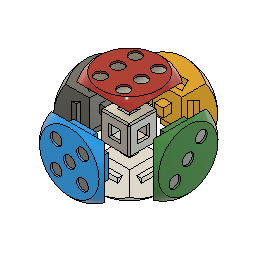
kostka v14 (Autodesk Fusion 360 design; units mm, degrees)
Autodesk Fusion 360 part; units mm, degrees
sketch "Sketch1" plane through (0, 0, 0) normal (0, 0, 1) x (1, 0, 0)
  line L0 (12, -12) -> (-12, -12)
  line L1 (-12, -12) -> (-12, 12)
  line L2 (-12, 12) -> (12, 12)
  line L3 (12, 12) -> (12, -12)
  line L4 (12, -12) -> (-12, 12) construction
  line L5 (-12, -12) -> (12, 12) construction
  line L6 (-5, -5) -> (5, -5)
  line L7 (5, -5) -> (5, 5)
  line L8 (5, 5) -> (-5, 5)
  line L9 (-5, 5) -> (-5, -5)
  line L10 (-5, -5) -> (5, 5) construction
  line L11 (5, -5) -> (-5, 5) construction
  dimension "d1" = 24
  dimension "d2" = 24
  dimension "d6" = 10
  dimension "d7" = 10
  constraint horizontal L0
  constraint perpendicular L0 L1
  constraint parallel L0 L2
  constraint parallel L1 L3
  constraint coincident L4 origin
  constraint coincident L5 origin
  constraint horizontal L6
  constraint perpendicular L6 L7
  constraint parallel L6 L8
  constraint parallel L7 L9
  constraint coincident L10 origin
  constraint coincident L11 origin
  measures "d1" distance of L1.end L2.end
  measures "d2" distance of L0.end L1.end
  measures "d6" distance of L7.end L8.end
  measures "d7" distance of L6.end L7.end
extrude "Extrude1" add sketch "Sketch1" along normal mid plane 24 makes body 1
ref_plane "WorkPlane1" through (-12, -12, -12) normal (0.707107, -0.707107, 0) x (0.707107, 0.707107, 0)
ref_plane "WorkPlane2" through (12, -12, -12) normal (-0.707107, -0.707107, 0) x (0.707107, -0.707107, 0)
ref_plane "WorkPlane3" through (12, -12, -12) normal (0, -0.707107, 0.707107) x (1, 0, 0)
ref_plane "WorkPlane4" through (12, -12, 12) normal (0, 0.707107, 0.707107) x (-1, 0, 0)
sphere "SpherePrimitive1" add diameter 31.5 placed x (1, 0, 0) y (0, 1, 0) z (0, 0, 1) at (0, 0, 0) separate body makes body 2
combine "Combine1" operation intersect target body 1 tool bodies 2 keep tools
split "Split1" by plane through (12, -12, 12) normal (0, 0.707107, 0.707107) bodies 1 makes body 3 at (9.4212, 10.076, -7.6011)
split "Split2" by plane through (12, -12, -12) normal (0, -0.707107, 0.707107) bodies 1 makes body 4 at (-2.4987, -12, 0.2541)
split "Split3" by plane through (-12, -12, -12) normal (0.707107, -0.707107, 0) bodies 4 makes body 5 at (-2.4987, -12, 0.2541)
split "Split4" by plane through (12, -12, -12) normal (-0.707107, -0.707107, 0) bodies 5 makes body 6 at (-2.4987, -12, 0.2541)
ref_plane "WorkPlane5" through (0, -8, 0) normal (0, 1, 0) x (-1, 0, 0)
sketch "Sketch7" plane through (0, -8, 0) normal (0, 1, 0) x (1, 0, 0)
  line L0 (4, -8) -> (-4, -8)
  line L1 (-4, -8) -> (-4, -6)
  line L2 (-4, -6) -> (4, -6)
  line L3 (4, -6) -> (4, -8)
  line L4 (4, -8) -> (-4, -6) construction
  line L5 (-4, -8) -> (4, -6) construction
  line L6 (6, -4) -> (6, 4)
  line L7 (6, 4) -> (8, 4)
  line L8 (8, 4) -> (8, -4)
  line L9 (8, -4) -> (6, -4)
  line L10 (4, 6) -> (-4, 6)
  line L11 (-4, 6) -> (-4, 8)
  line L12 (-4, 8) -> (4, 8)
  line L13 (4, 8) -> (4, 6)
  line L14 (-6, 4) -> (-6, -4)
  line L15 (-6, -4) -> (-8, -4)
  line L16 (-8, -4) -> (-8, 4)
  line L17 (-8, 4) -> (-6, 4)
  line L18 (1.5, -1.5) -> (-1.5, -1.5)
  line L19 (-1.5, -1.5) -> (-1.5, 1.5)
  line L20 (-1.5, 1.5) -> (1.5, 1.5)
  line L21 (1.5, 1.5) -> (1.5, -1.5)
  line L22 (1.5, -1.5) -> (-1.5, 1.5) construction
  line L23 (-1.5, -1.5) -> (1.5, 1.5) construction
  point P0 (0, -7)
  dimension "d9" = 8
  dimension "d10" = 2
  dimension "d12" = 360
  dimension "d15" = 7
  dimension "d70" = 3
  dimension "d71" = 3
  constraint horizontal L0
  constraint perpendicular L0 L1
  constraint parallel L0 L2
  constraint parallel L1 L3
  constraint coincident L4 P0
  constraint coincident L5 P0
  constraint horizontal L18
  constraint perpendicular L18 L19
  constraint parallel L18 L20
  constraint parallel L19 L21
  constraint coincident L22 origin
  constraint coincident L23 origin
  measures "d9" distance of L1.end L2.end
  measures "d10" distance of L0.end L1.end
  measures "d15" distance of origin P0
  measures "d70" distance of L19.end L20.end
  measures "d71" distance of L18.end L19.end
extrude "Extrude4" add sketch "Sketch7" along normal blind 6 contours L18 L19 L20 L21 bodies 6
extrude "Extrude3" cut sketch "Sketch7" along normal through all contours L10 L11 L12 L13 | L14 L15 L16 L17 bodies 6
extrude "Extrude2" add sketch "Sketch7" along normal blind 1.5 contours L0 L1 L2 L3 | L6 L7 L8 L9 bodies 6
move_face "OffsetFaces1" offset -0.03 4 faces at (9.037, -9.037, -0.3588) (-0.3588, -9.037, -9.037) (-9.037, -9.037, 0.3588) (0.3588, -9.037, 9.037) on bodies 6
move_face "OffsetFaces3" offset -0.05 8 faces at (-6.6525, -8, 1.3333) (-6.7391, -7.5, 4) (-6, -7.5, -1.3333) (-6.7391, -7.5, -4) (1.3333, -7.5, -6) (1.3333, -8, -7.305) (4, -7.5, -6.7391) (-4, -7.5, -6.7391) on bodies 6
copy_body "CopyPasteBodies1" bodies 6 makes body 7
move_body "Move1" bodies 7 to x (1, 0, 0) y (0, -1, 0) z (0, 0, -1) at (0, 0, 0)
copy_body "CopyPasteBodies2" bodies 6 makes body 8
move_body "Move2" bodies 8 to x (0, -1, 0) y (0, 0, -1) z (1, 0, 0) at (0, 0, 0)
copy_body "CopyPasteBodies3" bodies 6 makes body 9
move_body "Move3" bodies 9 to x (1, 0, 0) y (0, 0, 1) z (0, -1, 0) at (0, 0, 0)
copy_body "CopyPasteBodies4" bodies 6 makes body 10
move_body "Move4" bodies 10 to x (0, -1, 0) y (1, 0, 0) z (0, 0, 1) at (0, 0, 0)
copy_body "CopyPasteBodies5" bodies 6 makes body 11
move_body "Move5" bodies 11 to x (0, 1, 0) y (-1, 0, 0) z (0, 0, 1) at (0, 0, 0)
copy_body "Body->Comp1" bodies 6 removing the originals makes body 12 in component "No1"
copy_body "Body->Comp2" bodies 7 removing the originals makes body 13 in component "No6"
copy_body "Body->Comp3" bodies 8 removing the originals makes body 14 in component "No5"
copy_body "Body->Comp4" bodies 9 removing the originals makes body 15 in component "No2"
copy_body "Body->Comp5" bodies 10 removing the originals makes body 16 in component "No4"
copy_body "Body->Comp6" bodies 11 removing the originals makes body 17 in component "No3"
move_face "MoveFace1" to x (1, 0, 0) y (0, 0, -1) z (0, 1, 0) at (0, 0, 0) 1 faces at (12, -1.0078, -1.1876) on bodies 17 in component "No3"
sketch "Sketch1 (2)" plane through (0, 12, 0) normal (0, 1, 0) x (-1, 0, 0) in component "No6"
  circle A0 centre (0, 0) radius 10.2011
  circle A1 centre (0, 0) radius 2 construction
  circle A2 centre (-6, -4) radius 2
  circle A3 centre (0, -4) radius 2
  circle A4 centre (6, -4) radius 2
  circle A5 centre (-6, 4) radius 2
  circle A6 centre (0, 4) radius 2
  circle A7 centre (6, 4) radius 2
  dimension "d27" = 4
  dimension "d30" = 6
  dimension "d31" = 4
  constraint coincident A0.centre A1.centre
  measures "d27" diameter of A1
extrude "Extrude2'" cut sketch "Sketch1 (2)" against normal blind 0.6 contours A2 | A3 | A4 | A5 | A6 | A7 bodies 13 in component "No6"
sketch "Sketch1 (3)" plane through (0, -12, 0) normal (0, -1, 0) x (1, 0, 0) in component "No1"
  circle A0 centre (0, 0) radius 10.2011
  circle A1 centre (0, 0) radius 2
  dimension "d37" = 4
  constraint coincident A0.centre A1.centre
  measures "d37" diameter of A1
extrude "Extrude1'" cut sketch "Sketch1 (3)" against normal blind 0.6 contours A1 bodies 12 in component "No1"
sketch "Sketch1 (4)" plane through (0, 0, 12) normal (0, 0, 1) x (1, 0, 0) in component "No5"
  circle A0 centre (0, 0) radius 10.2011
  circle A1 centre (0, 0) radius 2
  circle A2 centre (-4.5255, 4.5255) radius 2
  line L0 (0, 0) -> (-6.7167, 6.7167) construction
  line L1 (0, 0) -> (-11, 0) construction
  circle A3 centre (-4.5255, -4.5255) radius 2
  circle A4 centre (4.5255, -4.5255) radius 2
  circle A5 centre (4.5255, 4.5255) radius 2
  dimension "d40" = 4
  dimension "d41" = 4
  dimension "d42" = 6.4
  dimension "d43" = 45
  dimension "d45" = 360
  constraint coincident A0.centre A1.centre
  constraint coincident A2.centre L0
  constraint coincident L0 A0.centre
  constraint horizontal L1
  measures "d40" diameter of A1
  measures "d41" diameter of A2
  measures "d42" distance of A0.centre A2.centre
  measures "d43" angle of L0 L1
extrude "Extrude1''" cut sketch "Sketch1 (4)" against normal blind 0.6 contours A1 | A2 | A3 | A4 | A5 bodies 14 in component "No5"
sketch "Sketch1 (5)" plane through (0, 0, -12) normal (0, 0, -1) x (-1, 0, 0) in component "No2"
  circle A0 centre (0, 0) radius 10.2011
  circle A1 centre (-4.5255, 4.5255) radius 2
  line L0 (-4.5255, 4.5255) -> (0, 0) construction
  line L1 (0, 0) -> (-10.2011, 0) construction
  circle A2 centre (4.5255, -4.5255) radius 2
  dimension "d48" = 4
  dimension "d49" = 6.4
  dimension "d50" = 45
  dimension "d52" = 360
  constraint coincident A1.centre L0.start
  constraint coincident A0.centre L0.end
  constraint coincident A0 L1.end
  constraint horizontal L1
  measures "d48" diameter of A1
  measures "d49" distance of A1.centre A0.centre
  measures "d50" angle of L0 L1
extrude "Extrude1'''" cut sketch "Sketch1 (5)" against normal blind 0.6 contours A1 | A2 bodies 15 in component "No2"
sketch "Sketch1 (6)" plane through (-12, 0, 0) normal (-1, 0, 0) x (0, 0, 1) in component "No4"
  circle A0 centre (0, 0) radius 10.2011
  circle A1 centre (-4.5255, -4.5255) radius 2
  line L0 (-4.5255, -4.5255) -> (0, 0) construction
  line L1 (0, 0) -> (0, -10.2011) construction
  circle A2 centre (4.5255, -4.5255) radius 2
  circle A3 centre (4.5255, 4.5255) radius 2
  circle A4 centre (-4.5255, 4.5255) radius 2
  dimension "d55" = 4
  dimension "d56" = 45
  dimension "d57" = 6.4
  dimension "d59" = 360
  constraint coincident A1.centre L0.start
  constraint coincident A0.centre L0.end
  constraint coincident A0 L1.end
  constraint vertical L1
  measures "d55" diameter of A1
  measures "d56" angle of L0 L1
  measures "d57" distance of A1.centre A0.centre
extrude "Extrude1''''" cut sketch "Sketch1 (6)" against normal blind 0.6 contours A1 | A2 | A3 | A4 bodies 16 in component "No4"
sketch "Sketch1 (7)" plane through (12, 0, 0) normal (1, 0, 0) x (0, 0, -1) in component "No3"
  circle A0 centre (0, 0) radius 10.2011
  circle A1 centre (4.5255, -4.5255) radius 2
  line L0 (4.5255, -4.5255) -> (0, 0) construction
  line L1 (0, 0) -> (10.2011, 0) construction
  circle A2 centre (-4.5255, 4.5255) radius 2
  circle A3 centre (0, 0) radius 2
  dimension "d62" = 4
  dimension "d63" = 6.4
  dimension "d64" = 45
  dimension "d66" = 360
  dimension "d67" = 4
  constraint coincident A1.centre L0.start
  constraint coincident A0.centre L0.end
  constraint coincident A0 L1.end
  constraint horizontal L1
  measures "d62" diameter of A1
  measures "d63" distance of A1.centre A0.centre
  measures "d64" angle of L0 L1
  measures "d67" diameter of A3
extrude "Extrude1'''''" cut sketch "Sketch1 (7)" against normal blind 0.6 contours A1 | A2 | A3 bodies 17 in component "No3"
sketch "Internal brick" plane through (0, 0, 0) normal (0, 0, 1) x (1, 0, 0)
  line L0 (4.975, -4.975) -> (-4.975, -4.975)
  line L1 (-4.975, -4.975) -> (-4.975, 4.975)
  line L2 (-4.975, 4.975) -> (4.975, 4.975)
  line L3 (4.975, 4.975) -> (4.975, -4.975)
  line L4 (4.975, -4.975) -> (-4.975, 4.975) construction
  line L5 (-4.975, -4.975) -> (4.975, 4.975) construction
  line L6 (1.525, -1.525) -> (-1.525, -1.525)
  line L7 (-1.525, -1.525) -> (-1.525, 1.525)
  line L8 (-1.525, 1.525) -> (1.525, 1.525)
  line L9 (1.525, 1.525) -> (1.525, -1.525)
  line L10 (1.525, -1.525) -> (-1.525, 1.525) construction
  line L11 (-1.525, -1.525) -> (1.525, 1.525) construction
  dimension "d74" = 9.95
  dimension "d75" = 9.95
  dimension "d76" = 3.05
  dimension "d77" = 3.05
  constraint horizontal L0
  constraint perpendicular L0 L1
  constraint parallel L0 L2
  constraint parallel L1 L3
  constraint coincident L4 origin
  constraint coincident L5 origin
  constraint horizontal L6
  constraint perpendicular L6 L7
  constraint parallel L6 L8
  constraint parallel L7 L9
  constraint coincident L10 origin
  constraint coincident L11 origin
  measures "d74" distance of L1.end L2.end
  measures "d75" distance of L0.end L1.end
  measures "d76" distance of L7.end L8.end
  measures "d77" distance of L6.end L7.end
extrude "Extrude1''''''" add sketch "Internal brick" along normal mid plane 9.95 separate body makes body 18 in component "Internal brick"
sketch "Sketch1 (8)" plane through (4.975, 0, 0) normal (1, 0, 0) x (0, 0, -1) in component "Internal brick"
  line L0 (4.975, 4.975) -> (-4.975, 4.975)
  line L1 (-4.975, 4.975) -> (-4.975, -4.975)
  line L2 (-4.975, -4.975) -> (4.975, -4.975)
  line L3 (4.975, -4.975) -> (4.975, 4.975)
  line L4 (1.525, -1.525) -> (-1.525, -1.525)
  line L5 (-1.525, -1.525) -> (-1.525, 1.525)
  line L6 (-1.525, 1.525) -> (1.525, 1.525)
  line L7 (1.525, 1.525) -> (1.525, -1.525)
  line L8 (1.525, -1.525) -> (-1.525, 1.525) construction
  line L9 (-1.525, -1.525) -> (1.525, 1.525) construction
  dimension "d82" = 3.05
  dimension "d83" = 3.05
  constraint horizontal L4
  constraint perpendicular L4 L5
  constraint parallel L4 L6
  constraint parallel L5 L7
  constraint coincident L8 origin
  constraint coincident L9 origin
  measures "d82" distance of L5.end L6.end
  measures "d83" distance of L4.end L5.end
extrude "Extrude2''" cut sketch "Sketch1 (8)" against normal through all contours L4 L5 L6 L7 bodies 18 in component "Internal brick"
sketch "Sketch2" plane through (0, 4.975, 0) normal (0, 1, 0) x (-1, 0, 0) in component "Internal brick"
  line L0 (4.975, -4.975) -> (4.975, 4.975)
  line L1 (4.975, 4.975) -> (-4.975, 4.975)
  line L2 (-4.975, 4.975) -> (-4.975, -4.975)
  line L3 (-4.975, -4.975) -> (4.975, -4.975)
  line L4 (-1.525, 1.525) -> (1.525, 1.525)
  line L5 (1.525, 1.525) -> (1.525, -1.525)
  line L6 (1.525, -1.525) -> (-1.525, -1.525)
  line L7 (-1.525, -1.525) -> (-1.525, 1.525)
  line L8 (-1.525, 1.525) -> (1.525, -1.525) construction
  line L9 (1.525, 1.525) -> (-1.525, -1.525) construction
  dimension "d85" = 3.05
  dimension "d86" = 3.05
  constraint horizontal L4
  constraint perpendicular L4 L5
  constraint parallel L4 L6
  constraint parallel L5 L7
  constraint coincident L8 origin
  constraint coincident L9 origin
  measures "d85" distance of L5.end L6.end
  measures "d86" distance of L4.end L5.end
extrude "Extrude3'" cut sketch "Sketch2" against normal through all contours L4 L5 L6 L7 bodies 18 in component "Internal brick"
chamfer "Chamfer1" distance 0.5 angle 45 6 faces at (-4.975, -0.5083, 3.825) (3.825, -4.975, 0.5083) (4.975, 3.825, -0.5083) (-3.825, 4.975, -0.5083) (-3.825, 0.5083, 4.975) (-3.825, 0.5083, -4.975) on bodies 18 in component "Internal brick"
component "No1" placed x (1, 0, 0) y (0, 1, 0) z (0, 0, 1) at (0, 0, 0)
component "No6" placed x (0, 0, -1) y (0, 1, 0) z (1, 0, 0) at (0, 7, 0)
component "No5" placed x (0, 1, 0) y (-1, 0, 0) z (0, 0, 1) at (0.248, 2.9321, 8.9569)
component "No2" placed x (0, -1, 0) y (1, 0, 0) z (0, 0, 1) at (1.7077, 4.3511, -6.2577)
component "No4" placed x (1, 0, 0) y (0, 1, 0) z (0, 0, 1) at (-6.3925, 1.8766, -2.5928)
component "No3" placed x (1, 0, 0) y (0, 0, -1) z (0, 1, 0) at (7.9702, 3.0356, -0.1204)
component "Internal brick" placed x (1, 0, 0) y (0, 1, 0) z (0, 0, 1) at (0, 0, 0)
hidden bodies 1 2 3 4 5
equation "d = 4 mm" comment "Prumer dirky"
equation "d27 = d"
equation "d30 = d * 1.5"
equation "d31 = d * 1"
equation "h = 0.6 mm" comment "Hloubka dirky"
equation "d35 = -h"
equation "d37 = d"
equation "d38 = -h"
equation "d40 = d"
equation "d41 = d"
equation "d42 = d * 1.6"
equation "d46 = -h"
equation "d48 = d"
equation "d49 = d * 1.6"
equation "d53 = -h"
equation "d55 = d"
equation "d57 = d * 1.6"
equation "d60 = -h"
equation "d62 = d"
equation "d63 = d * 1.6"
equation "d67 = d"
equation "d68 = -h"
equation "d75 = a"
equation "d77 = b"
equation "a = 9.95 mm" comment "Hrana vnitřní kostky"
equation "b = 3.05 mm" comment "Velikost vnitřního rozměru kostky"
equation "d80 = a"
equation "d82 = b"
equation "d83 = b"
equation "d85 = b"
equation "d86 = b"
named bodies: "No1", "Strana", "No6", "Strana (1)", "No5", "Strana (2)", "No2", "Strana (3)", "No4", "Strana (4)", "No3", "Internal brick"
